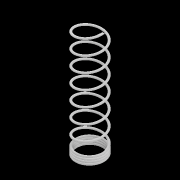
# Autodesk Inventor part: 螺旋鉤子
Saved by Autodesk Inventor 2020 (Build 240168000, 168)
## iProperties
Created: 2021-04-09
Part Number: 螺旋鉤子
Material: 一般
Document SubType Name: Modeling
Designer: 88690
Density: 1 g/cm^3
Appearance: 預設
Author: 88690
Autodesk Inventor part; units mm, degrees
ref_plane "YZ Plane" through (0, 0, 0) normal (1, 0, 0) x (0, 1, 0)
ref_plane "XZ Plane" through (0, 0, 0) normal (0, 1, 0) x (-1, 0, 0)
sketch "草圖1" plane through (0, 0, 0) normal (0, 0, 1) x (1, 0, 0)
  line L0 (-17.3172, 0) -> (17.3172, 0) construction
  line L1 (0, 0) -> (0, 500)
  circle A0 centre (65, 5) radius 5
  dimension "d0" = 10
  dimension "d1" = 130
  dimension "d2" = 500
  constraints: 4 end point, 1 centre point, 1 coincident, 1 horizontal, 1 midpoint, 1 tangent, 1 vertical
  measures "d0" diameter of A0
  measures "d1" diameter of A0.centre L1
  measures "d2" distance of L1.start L1.end
coil "螺旋3" sketch "草圖1" operation add axis through (0, 0, 0) along (0, 1, 0) pitch 71.4286 turns 7 hand right
sketch "草圖4" plane through (65, 5, 0) normal (0, 0, 1) x (1, 0, 0)
  circle A0 centre (0, 0) radius 5 projected
  circle A1 centre (0, 500) radius 5 construction
  line L0 (-74.0803, -5) -> (-55.9197, -5) construction
  line L1 (-65, -5) -> (-65, -45)
  circle A2 centre (0, 0) radius 5 projected
  circle A3 centre (0, 500) radius 5 construction
  point P0 (-135, 464.2857)
  point P1 (5, 428.5714)
  point P2 (-135, 392.8571)
  point P3 (5, 357.1429)
  point P4 (-135, 321.4286)
  point P5 (5, 285.7143)
  point P6 (-135, 250)
  point P7 (5, 214.2857)
  point P8 (-135, 178.5714)
  point P9 (5, 142.8571)
  point P10 (-135, 107.1429)
  point P11 (5, 71.4286)
  point P12 (-135, 35.7143)
  point P13 (5, 62.5)
  point P14 (-135, 31.25)
  point P15 (-135, 464.2857)
  point P16 (5, 428.5714)
  point P17 (-135, 392.8571)
  point P18 (5, 357.1429)
  point P19 (-135, 321.4286)
  point P20 (5, 285.7143)
  point P21 (-135, 250)
  point P22 (5, 214.2857)
  point P23 (-135, 178.5714)
  point P24 (5, 142.8571)
  point P25 (-135, 107.1429)
  point P26 (5, 71.4286)
  point P27 (-135, 35.7143)
  point P28 (5, 62.5)
  point P29 (-135, 31.25)
  dimension "d30" = 40
  constraints: 4 end point, 2 coincident, 1 horizontal, 1 midpoint, 1 vertical, 1 vertical alignment, 24 other
  measures "d30" distance of L1.start L1.end
coil "螺旋4" sketch "草圖4" operation add axis through (0, 0, 0) along (0, -1, 0) pitch 10.5263 turns 3.8 hand right
sketch "草圖5" plane through (0, 0, 0) normal (0, 0, 1) x (1, 0, 0)
  arc A0 (60, 5) -> (70, 5) centre (65, 5) ccw construction
  arc A1 (70, 5) -> (60, 5) centre (65, 5) ccw construction
  circle A2 centre (65, 505) radius 5 construction
  line L0 (102.7518, -35) -> (-232.7518, -35)
  line L1 (-232.7518, -35) -> (-232.7518, -231.6362)
  line L2 (-232.7518, -231.6362) -> (102.7518, -231.6362)
  line L3 (102.7518, -231.6362) -> (102.7518, -35)
  line L4 (259.9698, 505) -> (-129.9698, 505)
  line L5 (-129.9698, 505) -> (-129.9698, 679.4174)
  line L6 (-129.9698, 679.4174) -> (259.9698, 679.4174)
  line L7 (259.9698, 679.4174) -> (259.9698, 505)
  point P0 (0, 0)
  point P1 (-70, -31.8421)
  point P2 (70, -26.5789)
  point P3 (-70, -21.3158)
  point P4 (-70, -22.7778)
  point P5 (70, -17.2222)
  point P6 (-70, -11.6667)
  point P7 (70, -6.1111)
  point P8 (-70, -0.5556)
  point P9 (-70, 469.2857)
  point P10 (70, 433.5714)
  point P11 (-70, 397.8571)
  point P12 (70, 362.1429)
  point P13 (-70, 326.4286)
  point P14 (70, 290.7143)
  point P15 (-70, 255)
  point P16 (70, 219.2857)
  point P17 (-70, 183.5714)
  point P18 (70, 147.8571)
  point P19 (-70, 112.1429)
  point P20 (70, 76.4286)
  point P21 (-70, 40.7143)
  point P22 (70, 67.5)
  point P23 (-70, 36.25)
  point P24 (-65, -35)
  point P25 (65, 505)
  point P26 (-65, -35)
  point P27 (70, -16.0526)
  point P28 (-70, -10.7895)
  point P29 (70, -5.5263)
  point P30 (-70, -0.2632)
  constraints: 16 end point, 4 parallel, 2 coincident, 2 horizontal, 2 midpoint, 2 perpendicular, 20 other
extrude "擠出2" cut sketch "草圖5" along normal through all both and the other way through all
sketch "草圖12" plane through (0, 0, 0) normal (1, 0, 0) x (0, 1, 0)
  line L0 (-35, -69.9722) -> (-35, -60.0278) construction
  line L1 (487.1429, 70) -> (487.1429, 60) construction
  line L2 (415.7143, 70) -> (415.7143, 60) construction
  line L3 (487.1429, 65) -> (415.7143, 65) construction
  line L4 (451.4286, 65) -> (451.4286, -70) construction
  point P0 (0, 0)
  point P1 (-34.4737, -70)
  point P2 (-29.2105, 70)
  point P3 (-23.9474, -70)
  point P4 (-18.6842, 70)
  point P5 (-13.4211, -70)
  point P6 (-8.1579, 70)
  point P7 (-2.8947, -70)
  point P8 (2.3684, 70)
  point P9 (451.4286, -70)
  point P10 (380, -70)
  point P11 (344.2857, 70)
  point P12 (308.5714, -70)
  point P13 (272.8571, 70)
  point P14 (237.1429, -70)
  point P15 (201.4286, 70)
  point P16 (165.7143, -70)
  point P17 (130, 70)
  point P18 (94.2857, -70)
  point P19 (58.5714, 70)
  point P20 (22.8571, -70)
  constraints: 21 other
ref_plane "工作平面1" through (0, 451.4286, 65) normal (0, -1, 0) x (1, 0, 0)
sketch "草圖7" plane through (21.6312, -35, -66.574) normal (0, -1, 0) x (-0.309, 0, 0.9511)
  circle A0 centre (70, 0) radius 55
  circle A1 centre (70, 0) radius 70
  circle A2 centre (70, 0) radius 80
  point P0 (70, 0)
  dimension "d41" = 110
  dimension "d42" = 140
  dimension "d43" = 160
  constraints: 3 centre point, 3 coincident
  measures "d41" diameter of A0
  measures "d42" diameter of A1
  measures "d43" diameter of A2
sketch "草圖8" plane through (0, -35, 0) normal (0, -1, 0) x (1, 0, 0)
  circle A0 centre (0, 0) radius 80 projected
  point P0 (0, 0)
sketch "草圖9" plane through (0, -45, 0) normal (0, -1, 0) x (1, 0, 0)
  circle A0 centre (0, 0) radius 25
  point P0 (0, 0)
  dimension "d48" = 50
  constraints: 1 centre point, 1 coincident
  measures "d48" diameter of A0
equation "\"d23\" = d2"
equation "\"d32\" = d30"
